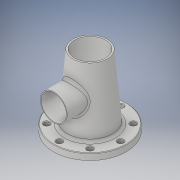
# Autodesk Inventor part: Součást12
Saved by Autodesk Inventor 2019 (Build 230136000, 136)
## iProperties
Created: 2019-11-25
Part Number: Součást12
Material: Všeobecné
Document SubType Name: Modeling
Designer: hynek
Density: 1 g/cm^3
Appearance: Výchozí
Author: hynek
Autodesk Inventor part; units mm, degrees
ref_plane "YZ Plane" through (0, 0, 0) normal (1, 0, 0) x (0, 1, 0)
ref_plane "XZ Plane" through (0, 0, 0) normal (0, 1, 0) x (-1, 0, 0)
sketch "Náčrt1" plane through (0, 0, 0) normal (0, 0, 1) x (1, 0, 0)
  line L0 (-40.537, 0) -> (-67.5, 0)
  line L1 (-67.5, 0) -> (-67.5, 12)
  line L2 (-67.5, 12) -> (-42.4986, 12)
  line L3 (-42.4986, 12) -> (-32, 132)
  line L4 (-32, 132) -> (-28.9885, 132)
  line L5 (-28.9885, 132) -> (-40.537, 0)
  line L6 (-81, 0) -> (13.5, 0) projected
  line L7 (0, -26.4) -> (0, 158.4) projected
  point P0 (0, 0)
  dimension "d0" = 12
  dimension "d1" = 132
  dimension "d2" = 32
  dimension "d4" = 3
  dimension "d5" = 67.5
  dimension "d6" = 5
  dimension "d7" = 0
  constraints: 12 end point, 2 horizontal, 2 perpendicular, 1 parallel
  measures "d0" distance between parallel lines of L2 L0
  measures "d1" distance between parallel lines of L6 L4
  measures "d2" distance from line of L3.end L7
  measures "d4" distance between parallel lines of L5 L3
  measures "d5" distance between parallel lines of L7 L1
  measures "d6" angle of L7 L5
  measures "d7" distance between parallel lines of L6 L0
revolve "Rotace1" add sketch "Náčrt1" angle 360 about axis through (0, -10, 0) along (0, 1, 0)
sketch "Náčrt2" plane through (0, 12, 0) normal (0, 1, 0) x (1, 0, 0)
  circle A0 centre (0, 0) radius 57 construction
  line L0 (0, 94.5) -> (0, -94.5) construction
  line L1 (-94.5, 0) -> (94.5, 0) construction
  circle A1 centre (0, 57) radius 5
  circle A2 centre (-40.3051, 40.3051) radius 5
  circle A3 centre (-57, 0) radius 5
  circle A4 centre (-40.3051, -40.3051) radius 5
  circle A5 centre (0, -57) radius 5
  circle A6 centre (40.3051, -40.3051) radius 5
  circle A7 centre (57, 0) radius 5
  circle A8 centre (40.3051, 40.3051) radius 5
  dimension "d9" = 114
  dimension "d11" = 10
  dimension "d14" = 360
  constraints: 8 centre point, 1 coincident, 1 point on line, 1 vertical alignment, 19 other
  measures "d11" diameter of A1
extrude "Vysunutí1" cut sketch "Náčrt2" against normal through all
chamfer "Zkosení1" distance 1 angle 45 9 edges at (-62, 12, 0) (-45.3051, 12, 40.3051) (-5, 12, 57) (35.3051, 12, 40.3051) (52, 12, 0) (35.3051, 12, -40.3051) (-5, 12, -57) (-45.3051, 12, -40.3051) (67.5, 12, 0)
ref_plane "Pracovní rovina1" through (0, 0, 67.5) normal (0, 0, 1) x (1, 0, 0)
sketch "Náčrt3" plane through (0, 0, 67.5) normal (0, 0, 1) x (1, 0, 0)
  line L0 (0, -26.4) -> (0, 158.4) construction
  line L1 (-94.5, 0) -> (94.5, 0) construction
  circle A0 centre (0, 72) radius 25
  point P0 (0, 0)
  dimension "d22" = 50
  dimension "d23" = 72
  constraints: 1 centre point, 1 point on line
  measures "d22" diameter of A0
  measures "d23" distance from line of L1 A0.centre
extrude "Vysunutí2" add sketch "Náčrt3" against normal up to next
sketch "Náčrt4" plane through (0, 72, 67.5) normal (0, 0, 1) x (1, 0, 0)
  circle A0 centre (0, 0) radius 25 projected
  circle A1 centre (0, 0) radius 23.5
  point P0 (0, -72)
  dimension "d27" = 47
  constraints: 1 centre point, 1 coincident
  measures "d27" diameter of A1
extrude "Vysunutí3" cut sketch "Náčrt4" against normal up to next contours A1
fillet "Zaoblení1" radius 5 2 edges at (-24.9752, 70.8872, 27.7671) (42.4986, 12, 0)
